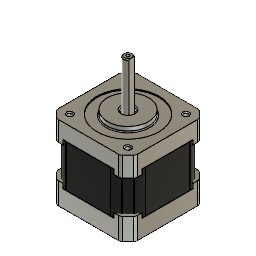
NEMA17_Stepper_Motor_F01 (Autodesk Fusion 360 design; units mm, degrees)
Autodesk Fusion 360 part; units mm, degrees
sketch "スケッチ1" plane through (0, 0, 0) normal (0, 0, 1) x (1, 0, 0)
  line L0 (21.15, 21.15) -> (-21.15, 21.15)
  line L1 (-21.15, 21.15) -> (-21.15, -21.15)
  line L2 (-21.15, -21.15) -> (21.15, -21.15)
  line L3 (21.15, -21.15) -> (21.15, 21.15)
  line L4 (21.15, 21.15) -> (-21.15, -21.15) construction
  line L5 (-21.15, 21.15) -> (21.15, -21.15) construction
  line L6 (16.92, 21.15) -> (21.15, 16.92)
  line L7 (21.15, -16.92) -> (16.92, -21.15)
  line L8 (-16.92, -21.15) -> (-21.15, -16.92)
  line L9 (-21.15, 16.92) -> (-16.92, 21.15)
  line L10 (14.38, 21.15) -> (21.15, 14.38)
  line L11 (21.15, -14.38) -> (14.38, -21.15)
  line L12 (-14.38, -21.15) -> (-21.15, -14.38)
  line L13 (-21.15, 14.38) -> (-14.38, 21.15)
  circle A0 centre (15.5, -15.5) radius 3
  circle A1 centre (15.5, 15.5) radius 3
  circle A2 centre (-15.5, 15.5) radius 3
  circle A3 centre (-15.5, -15.5) radius 3
  circle A4 centre (0, 0) radius 3.25
  circle A5 centre (0, 0) radius 2.5
  line L14 (13.62, 21.15) -> (13.62, 13.62)
  line L15 (13.62, 13.62) -> (21.15, 13.62)
  line L16 (-13.62, 13.62) -> (-13.62, 21.15)
  line L17 (-21.15, 13.62) -> (-13.62, 13.62)
  line L18 (-13.62, -13.62) -> (-21.15, -13.62)
  line L19 (-13.62, -21.15) -> (-13.62, -13.62)
  line L20 (13.62, -13.62) -> (13.62, -21.15)
  line L21 (21.15, -13.62) -> (13.62, -13.62)
  line L22 (2, 1.5) -> (2, -1.5)
  circle A6 centre (0, 0) radius 0.825
  dimension "d1" = 42.3
  dimension "d2" = 42.3
  dimension "d3" = 4.23
  dimension "d4" = 4.23
  dimension "d5" = 4.23
  dimension "d6" = 4.23
  dimension "d7" = 6.77
  dimension "d8" = 6.77
  dimension "d9" = 6.77
  dimension "d10" = 6.77
  dimension "d11" = 6
  dimension "d12" = 15.5
  dimension "d14" = 360
  dimension "d15" = 6.5
  dimension "d16" = 5
  dimension "d25" = 3.3
  dimension "d27" = 360
  dimension "d55" = 2
  dimension "d61" = 1.65
  measures "d3" distance of A4.centre
  measures "d4" distance of A4.centre
  measures "d5" distance of A4.centre
  measures "d6" distance of A4.centre
  measures "d7" distance of A4.centre
  measures "d8" distance of A4.centre
  measures "d9" distance of A4.centre
  measures "d10" distance of A4.centre
  measures "d11" diameter of A0
  measures "d12" distance of A4.centre
  measures "d15" diameter of A4
  measures "d16" diameter of A5
  measures "d25" distance of L14
  measures "d55" distance of A4.centre L22
  measures "d61" diameter of A6
extrude "押し出し1" add sketch "スケッチ1" along normal blind 9.2 contours L0 L3 L10 A1 L14 L15 | L0 L1 L2 L3 A0 A1 A2 A3 L14 L15 L16 L17 L18 L19 L20 L21 | L0 L1 L13 A2 L16 L17 | A1 L14 L15 | A1 L14 L15 | L2 L3 L11 A0 L20 L21 | A2 L16 L17 | A2 L16 L17 | A0 L20 L21 | A0 L20 L21 | L1 L2 L12 A3 L18 L19 | A3 L18 L19 | A3 L18 L19 makes body 1
extrude "押し出し2" add sketch "スケッチ1" along normal blind 11.7 contours L0 L3 L6 L10 | L0 L3 L10 A1 L14 L15 | L0 L1 L13 A2 L16 L17 | L2 L3 L11 A0 L20 L21 | L0 L1 L9 L13 | L2 L3 L7 L11 | L1 L2 L12 A3 L18 L19 | L1 L2 L8 L12 | A4 bodies 1
extrude "押し出し14" cut sketch "スケッチ1" along normal blind 2.1 contours A1 L14 L15 | A1 L14 L15 | A2 L16 L17 | A2 L16 L17 | A0 L20 L21 | A0 L20 L21 | A3 L18 L19 | A3 L18 L19 bodies 1
extrude "押し出し3" add sketch "スケッチ1" along normal blind 22.7 from surface at 9.2 separate body contours L0 L3 L10 A1 L14 L15 | L0 L1 L2 L3 A0 A1 A2 A3 L14 L15 L16 L17 L18 L19 L20 L21 | L0 L1 L13 A2 L16 L17 | A1 L14 L15 | A1 L14 L15 | L2 L3 L11 A0 L20 L21 | A2 L16 L17 | A2 L16 L17 | A0 L20 L21 | A0 L20 L21 | L1 L2 L12 A3 L18 L19 | A3 L18 L19 | A3 L18 L19 | A4 | A5 L22 | A5 L22 | A6 makes body 2
fillet "フィレット1" radius 6 8 edges at (21.15, -14.38, 20.55) (14.38, -21.15, 20.55) (-14.38, -21.15, 20.55) (-21.15, -14.38, 20.55) (-21.15, 14.38, 20.55) (-14.38, 21.15, 20.55) (14.38, 21.15, 20.55) (21.15, 14.38, 20.55) on bodies 2
extrude "押し出し4" add sketch "スケッチ1" against normal blind 8.1 from surface at 40 separate body contours L0 L3 L10 A1 L14 L15 | L0 L1 L2 L3 A0 A1 A2 A3 L14 L15 L16 L17 L18 L19 L20 L21 | L0 L1 L13 A2 L16 L17 | A1 L14 L15 | A1 L14 L15 | L2 L3 L11 A0 L20 L21 | A2 L16 L17 | A2 L16 L17 | A0 L20 L21 | A0 L20 L21 | L1 L2 L12 A3 L18 L19 | A3 L18 L19 | A3 L18 L19 | A4 | A5 L22 | A5 L22 | A6 makes body 3
extrude "押し出し5" add sketch "スケッチ1" against normal blind 10.6 from surface at 40 contours L0 L3 L6 L10 | L0 L3 L10 A1 L14 L15 | L0 L1 L13 A2 L16 L17 | A1 L14 L15 | L2 L3 L11 A0 L20 L21 | L0 L1 L9 L13 | A2 L16 L17 | L2 L3 L7 L11 | A0 L20 L21 | L1 L2 L12 A3 L18 L19 | L1 L2 L8 L12 | A3 L18 L19 picked at (16.2277, 16.3373) picked at (-16.1769, 16.3831) picked at (16.2277, -16.3373) picked at (-16.1769, -16.3831) bodies 3
fillet "フィレット2" radius 2 16 edges at (16.92, -21.15, 5.85) (21.15, -16.92, 5.85) (21.15, 16.92, 5.85) (16.92, 21.15, 5.85) (-21.15, 16.92, 5.85) (-16.92, 21.15, 5.85) (-21.15, -16.92, 5.85) (-16.92, -21.15, 5.85) (16.92, -21.15, 34.7) (21.15, -16.92, 34.7) (21.15, 16.92, 34.7) (16.92, 21.15, 34.7) (-16.92, 21.15, 34.7) (-21.15, 16.92, 34.7) (-16.92, -21.15, 34.7) (-21.15, -16.92, 34.7) on bodies 1 3
sketch "スケッチ2" plane through (0, 0, 40) normal (0, 0, 1) x (-1, 0, 0)
  arc A0 (21.15, 16.0916) -> (20.5642, 17.5058) centre (19.15, 16.0916) ccw
  line L0 (20.5642, 17.5058) -> (17.5058, 20.5642)
  arc A1 (17.5058, 20.5642) -> (16.0916, 21.15) centre (16.0916, 19.15) ccw
  line L1 (16.0916, 21.15) -> (-16.0916, 21.15)
  arc A2 (-16.0916, 21.15) -> (-17.5058, 20.5642) centre (-16.0916, 19.15) ccw
  line L2 (-17.5058, 20.5642) -> (-20.5642, 17.5058)
  arc A3 (-20.5642, 17.5058) -> (-21.15, 16.0916) centre (-19.15, 16.0916) ccw
  line L3 (-21.15, 16.0916) -> (-21.15, -16.0916)
  arc A4 (-21.15, -16.0916) -> (-20.5642, -17.5058) centre (-19.15, -16.0916) ccw
  line L4 (-20.5642, -17.5058) -> (-17.5058, -20.5642)
  arc A5 (-17.5058, -20.5642) -> (-16.0916, -21.15) centre (-16.0916, -19.15) ccw
  line L5 (-16.0916, -21.15) -> (16.0916, -21.15)
  arc A6 (16.0916, -21.15) -> (17.5058, -20.5642) centre (16.0916, -19.15) ccw
  line L6 (17.5058, -20.5642) -> (20.5642, -17.5058)
  arc A7 (20.5642, -17.5058) -> (21.15, -16.0916) centre (19.15, -16.0916) ccw
  line L7 (21.15, -16.0916) -> (21.15, 16.0916)
  circle A8 centre (-15.5, -15.5) radius 1.25
  circle A9 centre (15.5, -15.5) radius 1.25
  circle A10 centre (-15.5, 15.5) radius 1.25
  circle A11 centre (15.5, 15.5) radius 1.25
  circle A12 centre (0, 0) radius 16.5
  circle A13 centre (0, 0) radius 11
  circle A14 centre (0, 0) radius 3.25
  dimension "d35" = 2.5
  dimension "d36" = 2.5
  dimension "d37" = 2.5
  dimension "d38" = 2.5
  dimension "d42" = 33
  dimension "d43" = 22
  dimension "d49" = 6.5
  measures "d35" diameter of A8
  measures "d36" diameter of A9
  measures "d37" diameter of A10
  measures "d38" diameter of A11
  measures "d42" diameter of A12
  measures "d43" diameter of A13
  measures "d49" diameter of A14
extrude "押し出し6" cut sketch "スケッチ2" against normal blind 10 contours A8 | A9 | A10 | A11 bodies 2 3
chamfer "面取り1" distance 0.5 angle 45 4 edges at (-14.3346, 15.048, 40) (16.6654, 15.048, 40) (16.6654, -15.952, 40) (-14.3346, -15.952, 40) on bodies 3
extrude "押し出し7" cut sketch "スケッチ2" against normal blind 0.6 contours A12 bodies 3
extrude "押し出し8" add sketch "スケッチ2" along normal blind 2 contours A13 | A14 bodies 3
extrude "押し出し9" cut sketch "スケッチ2" along normal up to surface (2 mm away) contours A14 bodies 3
fillet "フィレット3" radius 0.5 2 edges at (10.2556, 3.9778, 39.4) (3.0301, -1.1753, 42) on bodies 3
extrude "押し出し10" cut sketch "スケッチ1" along normal blind 3 contours A4 bodies 1
extrude "押し出し11" add sketch "スケッチ1" along normal blind 64 from surface at 3 separate body contours A5 L22 | A6 picked at (1.6083, 0) makes body 4
extrude "押し出し12" cut sketch "スケッチ1" along normal blind 8 contours A6 bodies 4
sketch "スケッチ3" plane through (0, 0, 67) normal (0, 0, 1) x (-1, 0, 0)
  arc A0 (-2, -1.5) -> (-2, 1.5) centre (0, 0) ccw
  line L0 (-2, 1.5) -> (-2, -1.5)
  circle A1 centre (0, 0) radius 0.825
  dimension "d64" = 1.65
  measures "d64" diameter of A1
extrude "押し出し13" cut sketch "スケッチ3" against normal blind 5 contours A1 bodies 4
fillet "フィレット4" radius 0.5 2 edges at (-2.5, 0, 67) (-2.5, 0, 3) on bodies 4
sketch "スケッチ4" plane through (0, 0, 2.1) normal (0, 0, -1) x (1, 0, 0)
  circle A0 centre (15.5, 15.5) radius 3
  circle A1 centre (15.5, 15.5) radius 2.75
  dimension "d69" = 5.5
  measures "d69" diameter of A1
extrude "押し出し15" add sketch "スケッチ4" along normal blind 2 separate body contours A1 makes body 5
fillet "フィレット5" radius 1.5 1 edges at (12.9361, -14.5056, 0.1) on bodies 5
sketch "スケッチ5" plane through (0, 0, 0.1) normal (0, 0, -1) x (1, 0, 0)
  circle A0 centre (15.5, 15.5) radius 1.25
  line L0 (17.3, 15.65) -> (13.7, 15.65)
  line L1 (13.7, 15.65) -> (13.7, 15.35)
  line L2 (13.7, 15.35) -> (17.3, 15.35)
  line L3 (17.3, 15.35) -> (17.3, 15.65)
  line L4 (17.3, 15.65) -> (13.7, 15.35) construction
  line L5 (13.7, 15.65) -> (17.3, 15.35) construction
  line L6 (15.65, 17.3) -> (15.35, 17.3)
  line L7 (15.35, 17.3) -> (15.35, 13.7)
  line L8 (15.35, 13.7) -> (15.65, 13.7)
  line L9 (15.65, 13.7) -> (15.65, 17.3)
  line L10 (15.65, 17.3) -> (15.35, 13.7) construction
  line L11 (15.35, 17.3) -> (15.65, 13.7) construction
  dimension "d73" = 3.6
  dimension "d74" = 0.3
  dimension "d75" = 3.6
  dimension "d76" = 0.3
extrude "押し出し16" cut sketch "スケッチ5" against normal blind 1.2 contours A0 L0 L2 L9 | A0 L0 L2 L3 | A0 L0 L7 L9 | A0 L6 L7 L9 | L0 L2 L7 L9 | A0 L7 L8 L9 | A0 L2 L7 L9 | A0 L0 L2 L7 | A0 L0 L1 L2 bodies 5
pattern_circular "C パターン1" count 4 over 360 about axis through (0, 0, 1.75) along (0, 0, 1) of bodies 5 makes body 6 at (16.3345, 12.8875, 1.4508) makes body 7 at (-18.1125, 14.6655, 1.4508) makes body 8 at (-14.6655, -18.1125, 1.4508)
equation "d4 = d3"
equation "d5 = d3"
equation "d6 = d3"
equation "d8 = d7"
equation "d9 = d7"
equation "d10 = d7"
equation "d12 = ( 31 / 2 ) * 1 mm"
